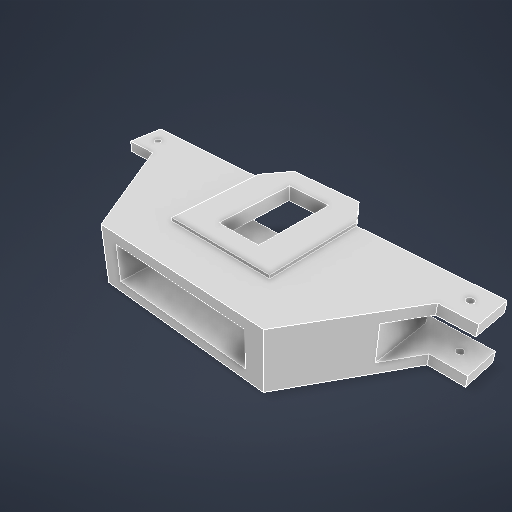
# Autodesk Inventor part: Front Bridge
Saved by Autodesk Inventor 2025 (Build 290162000, 162)
## iProperties
Created: 2024-05-23
Part Number: Front Bridge
Material: Generic
Document SubType Name: Modeling
Designer: DELL
Density: 1 g/cm^3
Appearance: Default
Mass: 43.2187 g
Surface Area: 102.411 cm^2
Volume: 43.2187 cm^3
Author: DELL
Autodesk Inventor part; units mm, degrees
ref_plane "YZ Plane" through (0, 0, 0) normal (1, 0, 0) x (0, 1, 0)
ref_plane "XZ Plane" through (0, 0, 0) normal (0, 1, 0) x (-1, 0, 0)
ref_plane "XY Plane" through (0, 0, 0) normal (0, 0, 1) x (1, 0, 0)
derived "Car_Plan.ipt"
sketch "Car_Sketch" plane through (0, 0, 0) normal (0, 1, 0) x (-1, 0, 0)
  line L0 (0, 0) -> (94, 0)
  line L1 (0, 0) -> (0, 105)
  line L2 (94, 0) -> (94, 105)
  line L3 (0, 105) -> (20, 105)
  line L4 (20, 105) -> (20, 190)
  line L5 (20, 190) -> (74, 190)
  line L6 (74, 190) -> (74, 105)
  line L7 (74, 105) -> (94, 105)
  line L8 (-5, 68) -> (-5, 0)
  line L9 (-5, 0) -> (-32, 0)
  line L10 (-32, 0) -> (-32, 68)
  line L11 (-32, 68) -> (-5, 68)
  line L12 (47, 190) -> (47, 0) construction
  line L13 (126, 68) -> (99, 68)
  line L14 (99, 68) -> (99, 0)
  line L15 (126, 0) -> (126, 68)
  line L16 (99, 0) -> (126, 0)
  line L17 (-5, 34) -> (99, 34) construction
  line L18 (0, 95) -> (94, 95) construction
  line L19 (-5, 190) -> (-32, 190)
  line L20 (-32, 122) -> (-5, 122)
  line L21 (-32, 190) -> (-32, 122)
  line L22 (-5, 122) -> (-5, 190)
  line L23 (-5, 156) -> (99, 156) construction
  line L24 (126, 122) -> (99, 122)
  line L25 (126, 190) -> (126, 122)
  line L26 (99, 190) -> (126, 190)
  line L27 (99, 122) -> (99, 190)
  line L28 (0, 156) -> (47, 34) construction
  line L29 (94, 156) -> (47, 34) construction
  line L30 (0, 156) -> (-174.2341, 34) construction
  line L31 (-5, 34) -> (-174.2341, 34) construction
  line L32 (8.9873, 132.6713) -> (47, 141.55) construction
  line L33 (85.0127, 132.6713) -> (47, 141.55) construction
sketch "Base" plane through (0, 0, 0) normal (0, 1, 0) x (-1, 0, 0)
  circle A0 centre (0, 156) radius 1
  circle A1 centre (94, 156) radius 1
  line L0 (-5, 161) -> (-5, 151)
  line L1 (-5, 151) -> (32, 151)
  line L2 (99, 151) -> (99, 161)
  line L3 (99, 161) -> (90, 161)
  line L4 (4, 161) -> (22, 190)
  line L5 (22, 190) -> (72, 190)
  line L6 (72, 190) -> (90, 161)
  line L7 (0, 156) -> (94, 156) construction
  line L8 (4, 161) -> (-5, 161)
  line L9 (40.95, 172.3) -> (53.05, 172.3)
  line L10 (53.05, 172.3) -> (53.05, 149.9)
  line L11 (53.05, 149.9) -> (40.95, 149.9)
  line L12 (40.95, 149.9) -> (40.95, 172.3)
  line L13 (47, 156) -> (47, 149.9) construction
  line L14 (32, 151) -> (37, 144)
  line L15 (37, 144) -> (57, 144)
  line L16 (57, 144) -> (62, 151)
  line L17 (47, 156) -> (47, 144) construction
  line L18 (32, 151) -> (62, 151)
  line L19 (62, 151) -> (99, 151)
  dimension "d130" = 2
  dimension "d131" = 2
  dimension "d132" = 5
  dimension "d134" = 5
  dimension "d136" = 5
  dimension "d137" = 5
  dimension "d138" = 4
  dimension "d139" = 5
  dimension "d140" = 34
  dimension "d143" = 50
  dimension "d168" = 16.3
  dimension "d169" = 12.1
  dimension "d170" = 22.4
  dimension "d173" = 6.05
  dimension "d174" = 12
  dimension "d175" = 20
  dimension "d176" = 15
  constraints: 40 end point, 11 perpendicular, 8 parallel, 3 equal length, 3 midpoint, 2 centre point, 2 coincident, 1 point on line
  measures "d130" diameter of A0
  measures "d131" diameter of A1
  measures "d132" distance from line of L0 L7.start
  measures "d134" distance from line of L1 point (0, 156)
  measures "d136" distance from line of L2 point (94, 156)
  measures "d137" distance from line of L3 point (94, 156)
  measures "d138" horizontal distance of L4.start point (0, 156)
  measures "d139" distance from line of L8 L7.start
  measures "d140" distance between parallel lines of L7 L5
  measures "d143" distance of L4.end L5.end
  measures "d168" distance from line of L9 L13.start
  measures "d169" distance of L10.end L11.end
  measures "d170" distance of L10.end L9.end
  measures "d173" distance between parallel lines of L12 L13
  measures "d174" distance of L17.end L13.start
  measures "d175" distance of L15.end L14.end
  measures "d176" distance from line of L17 L1.end
extrude "Base_Extrusion" add sketch "Base" along normal blind 16 contours L8 L4 L5 L6 L3 L2 L19 L18 L10 L9 L12 L1 L0 | L12 L9 L10 L18
sketch "Hole_For_Wheel_Anchor" plane through (5, 0, 151) normal (0, 0, -1) x (-1, 0, 0)
  line L0 (0, 0) -> (0, 16) projected
  line L1 (104, 0) -> (104, 16) projected
  line L2 (0, 13) -> (15, 13)
  line L3 (15, 13) -> (15, 3)
  line L4 (15, 3) -> (0, 3)
  line L5 (0, 16) -> (104, 16) construction
  line L6 (0, 0) -> (104, 0) construction
  line L7 (52, 16) -> (52, 0) construction
  line L8 (104, 13) -> (89, 13)
  line L9 (89, 13) -> (89, 3)
  line L10 (89, 3) -> (104, 3)
  point P0 (5, 0)
  dimension "d149" = 15
  dimension "d150" = 10
  dimension "d151" = 3
  constraints: 14 end point, 4 symmetric about line, 3 perpendicular, 2 midpoint, 2 point on line
  measures "d149" distance of L2.start L2.end
  measures "d150" distance of L3.end L2.end
  measures "d151" distance from line of L5 L2.end
extrude "Hole_For_Wheel_Anchor_Extrusion" cut sketch "Hole_For_Wheel_Anchor" against normal through all
chamfer "Chamfer_For_Wheel_Anchor" distance 4 angle 33 2 edges at (-10, 8, 151) (-84, 8, 151) measured on face at (-83.5, 8, 151) measured on face at (-10.5, 8, 151)
sketch "Hole_For_Servo_Arm" plane through (5, 0, 151) normal (0, 0, -1) x (-1, 0, 0)
  line L0 (27, 0) -> (27, 16) construction
  line L1 (77, 0) -> (77, 16) construction
  line L2 (0, 0) -> (104, 0) construction
  line L3 (0, 16) -> (104, 16) construction
  line L4 (32, 13) -> (32, 3)
  line L5 (32, 3) -> (72, 3)
  line L6 (72, 3) -> (72, 13)
  line L7 (72, 13) -> (32, 13)
  line L8 (52, 13) -> (52, 3) construction
  point P0 (5, 0)
  dimension "d173" = 6.05
  dimension "d160" = 25
  dimension "d161" = 40
  dimension "d162" = 10
  dimension "d163" = 3
  constraints: 10 end point, 3 perpendicular, 2 midpoint, 1 parallel
  measures "d160" distance between parallel lines of L0 L8
  measures "d161" distance of L5.end L4.end
  measures "d162" distance of L4.end L4.start
  measures "d163" distance between parallel lines of L2 L5
extrude "Hole_For_Servo_Arm_Extrusion" cut sketch "Hole_For_Servo_Arm" against normal through all
sketch "Servo_Extension" plane through (0, 16, 0) normal (0, 1, 0) x (1, 0, 0)
  line L0 (-32, -151) -> (-37, -144) projected
  line L1 (-32, -151) -> (-62, -151) projected
  line L2 (-57, -144) -> (-62, -151) projected
  line L3 (-37, -144) -> (-57, -144) projected
extrude "Servo_Extension_Extrusion" add sketch "Servo_Extension" against normal up to surface (3 mm away)
sketch "Hole_For_Servo" plane through (0, 16, 0) normal (0, 1, 0) x (1, 0, 0)
  line L0 (-40.95, -149.9) -> (-40.95, -172.3) projected
  line L1 (-53.05, -149.9) -> (-40.95, -149.9) projected
  line L2 (-53.05, -172.3) -> (-53.05, -149.9) projected
  line L3 (-40.95, -172.3) -> (-53.05, -172.3) projected
extrude "Hole_For_Servo_Extrusion" cut sketch "Hole_For_Servo" against normal up to surface (3 mm away)
sketch "Servo_Bump" plane through (0, 16, 0) normal (0, 1, 0) x (1, 0, 0)
  line L0 (-32, -151) -> (-37, -144) projected
  line L1 (-37, -144) -> (-57, -144) projected
  line L2 (-57, -144) -> (-62, -151) projected
  line L3 (-32, -151) -> (-32, -178.2)
  line L4 (-32, -178.2) -> (-62, -178.2)
  line L5 (-62, -178.2) -> (-62, -151)
  line L6 (-40.95, -149.9) -> (-40.95, -172.3) projected
  line L7 (-53.05, -149.9) -> (-40.95, -149.9) projected
  line L8 (-53.05, -172.3) -> (-53.05, -149.9) projected
  line L9 (-40.95, -172.3) -> (-53.05, -172.3) projected
  line L10 (-40.95, -149.9) -> (-53.05, -149.9) projected
  line L11 (-47, -149.9) -> (-47, -144) construction
  line L12 (-47, -172.3) -> (-47, -178.2) construction
  constraints: 10 end point, 4 midpoint, 2 parallel, 1 collinear, 1 perpendicular
extrude "Servo_Bump_Extrusion" add sketch "Servo_Bump" along normal blind 0.95
body "Solid3"
